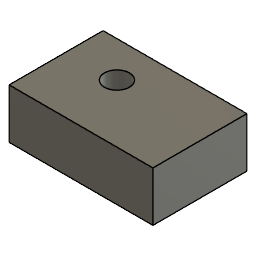
replay (Autodesk Fusion 360 design; units mm, degrees)
Autodesk Fusion 360 part; units mm, degrees
sketch "草图1" plane through (0, 0, 0) normal (0, 1, 0) x (1, 0, 0)
  line L0 (44, -40) -> (44, -6)
  line L1 (44, -6) -> (-8, -6)
  line L2 (-8, -6) -> (-8, -40)
  line L3 (-8, -40) -> (44, -40)
extrude "拉伸1" add sketch "草图1" along normal blind 18
sketch "草图2" plane through (0, 18, 0) normal (0, 1, 0) x (0, 0, 1)
  line L0 (40, -8) -> (40, 44)
  line L1 (40, 44) -> (6, 44)
  line L2 (6, 44) -> (6, -8)
  line L3 (6, -8) -> (40, -8)
  circle A0 centre (19, 10) radius 4.5
extrude "拉伸2" cut sketch "草图2" against normal through all contours A0
